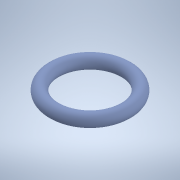
# Autodesk Inventor part: МПСТ Мазеудерживающее кольцо быстроходного вала
Saved by Autodesk Inventor 2022.1 (Build 261234020, 234B)
## iProperties
Created: 2021-12-16
Part Number: МПСТ Мазеудерживающее кольцо быстроходного вала
Material: Резина
Document SubType Name: Modeling
Designer: Алексанян Г.
Density: 0.93 g/cm^3
Appearance: Резина — синяя
Author: Алексанян Г.
Autodesk Inventor part; units mm, degrees
ref_plane "YZ Plane" through (0, 0, 0) normal (1, 0, 0) x (0, 1, 0)
ref_plane "XZ Plane" through (0, 0, 0) normal (0, 1, 0) x (-1, 0, 0)
ref_plane "XY Plane" through (0, 0, 0) normal (0, 0, 1) x (1, 0, 0)
sketch "Эскиз1" plane through (0, 0, 0) normal (0, 0, 1) x (1, 0, 0)
  line L0 (0, 33.3944) -> (0, -29.771)
  circle A0 centre (-20, 0) radius 3.5
  point P0 (0, 0)
  dimension "d0" = 7
  dimension "d1" = 40
  constraints: 2 end point, 1 centre point, 1 horizontal alignment, 1 vertical, 1 vertical alignment
  measures "d0" diameter of A0
  measures "d1" diameter of A0.centre L0
revolve "Вращение1" add sketch "Эскиз1" angle 360 about axis through (0, 33.3944, 0) along (0, -1, 0)
